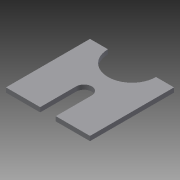
# Autodesk Inventor part: torchArm
Saved by Autodesk Inventor 2013 (Build 170138000, 138)
## iProperties
Created: 2012-12-09
Part Number: torchArm
Material: Generic
Document SubType Name: Modeling
Designer: Istvan
Density: 1 g/cm^3
Mass: 29.3071 g
Surface Area: 145.469 cm^2
Volume: 29.3071 cm^3
Author: Istvan
Autodesk Inventor part; units mm, degrees
ref_plane "YZ Plane" through (0, 0, 0) normal (1, 0, 0) x (0, 1, 0)
ref_plane "XZ Plane" through (0, 0, 0) normal (0, 1, 0) x (-1, 0, 0)
ref_plane "XY Plane" through (0, 0, 0) normal (0, 0, 1) x (1, 0, 0)
sketch "Sketch1" plane through (0, 0, 0) normal (0, 1, 0) x (-1, 0, 0)
  line L0 (0, 0) -> (19.05, 0)
  line L1 (44.45, 25.4) -> (44.45, 42.545)
  line L2 (36.195, 88.9) -> (0, 88.9)
  line L3 (0, 88.9) -> (0, 0)
  line L4 (36.195, 88.9) -> (16.9101, 88.9)
  line L5 (36.195, 50.8) -> (36.195, 88.9)
  arc A0 (36.195, 50.8) -> (44.45, 42.545) centre (44.45, 50.8) ccw
  line L6 (9.525, 0) -> (19.05, 0)
  line L7 (19.05, 0) -> (19.05, 0)
  line L8 (44.45, 25.4) -> (44.45, 25.4)
  arc A1 (44.45, 25.4) -> (19.05, 0) centre (44.45, 0) ccw
  dimension "d2" = 8.255
  dimension "d8" = 38.1
  dimension "d9" = 88.9
  dimension "d10" = 25.4
  dimension "d11" = 44.45
  constraints: 19 end point, 4 horizontal, 4 point on circle, 3 parallel, 3 tangent, 2 centre point, 2 perpendicular, 1 coincident, 1 midpoint, 1 point on line, 1 vertical, 3 other
  measures "d2" radius of A0
  measures "d8" distance of L2.start L5.start
  measures "d9" distance of L2.end L0.start
  measures "d10" radius of A1
  measures "d11" distance between parallel lines of L3 L1
extrude "Extrusion1" add sketch "Sketch1" along normal blind 4.7625
mirror "Mirror1" about plane through (-44.45, 0, 25.4) normal (-1, 0, 0)
body "Solid1"
